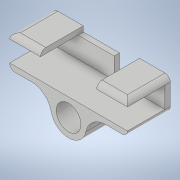
# Autodesk Inventor part: camera_holder
Saved by Autodesk Inventor 2020 (Build 240168000, 168)
## iProperties
Created: 2018-05-19
Part Number: camera_holder
Material: Generic
Document SubType Name: Modeling
Designer: stedrock
Density: 1 g/cm^3
Appearance: Default
Mass: 31.7935 g
Surface Area: 154.561 cm^2
Volume: 31.7935 cm^3
Author: stedrock
Autodesk Inventor part; units mm, degrees
ref_plane "YZ Plane" through (0, 0, 0) normal (1, 0, 0) x (0, 1, 0)
ref_plane "XZ Plane" through (0, 0, 0) normal (0, 1, 0) x (-1, 0, 0)
ref_plane "XY Plane" through (0, 0, 0) normal (0, 0, 1) x (1, 0, 0)
sketch "Sketch1" plane through (0, 0, 0) normal (0, 0, 1) x (1, 0, 0)
  line L0 (-44, -7.75) -> (44, -7.75)
  line L1 (44, -7.75) -> (44, 7.75)
  line L2 (44, 7.75) -> (-44, 7.75)
  line L3 (-44, 7.75) -> (-44, -7.75)
  line L4 (-44, -7.75) -> (44, 7.75) construction
  line L5 (44, -7.75) -> (-44, 7.75) construction
  line L6 (-44, -7.75) -> (44, -7.75)
  line L7 (44, -7.75) -> (44, -11.75)
  line L8 (44, -11.75) -> (-44, -11.75)
  line L9 (-44, -11.75) -> (-44, -7.75)
  line L10 (-44, 7.75) -> (-21, 7.75)
  line L11 (-21, 7.75) -> (-21, 11.75)
  line L12 (-21, 11.75) -> (-44, 11.75)
  line L13 (-44, 11.75) -> (-44, 7.75)
  line L14 (44, 7.75) -> (21, 7.75)
  line L15 (21, 7.75) -> (21, 11.75)
  line L16 (21, 11.75) -> (44, 11.75)
  line L17 (44, 11.75) -> (44, 7.75)
  line L18 (0, 0) -> (0, -41.0889) construction
  circle A0 centre (0, -21) radius 9.25
  circle A1 centre (0, -21) radius 13.25
  line L19 (-13.25, -21) -> (-13.25, -11.75)
  line L20 (-13.25, -11.75) -> (-9.4868, -11.75)
  line L21 (13.25, -11.75) -> (9.4868, -11.75)
  line L22 (13.25, -21) -> (13.25, -11.75)
  line L23 (13.25, -11.75) -> (9.4868, -11.75)
  line L24 (0, 0) -> (65.293, 0) construction
  line L25 (21, -7.75) -> (6, -7.75)
  line L26 (6, -7.75) -> (6, 7.75)
  line L27 (6, 7.75) -> (21, 7.75)
  line L28 (21, 7.75) -> (21, -7.75)
  line L29 (21, -7.75) -> (6, 7.75) construction
  line L30 (6, -7.75) -> (21, 7.75) construction
  point P0 (13.25, -21)
  point P1 (13.5, 0)
  dimension "d0" = 88
  dimension "d1" = 15.5
  dimension "d2" = 4
  dimension "d3" = 4
  dimension "d4" = 23
  dimension "d5" = 23
  dimension "d6" = 18.5
  dimension "d7" = 26.5
  dimension "d8" = 90
  dimension "d19" = 15
  dimension "d20" = 15.5
  dimension "d21" = 23
  constraints: 62 end point, 10 parallel, 6 horizontal, 6 point on line, 5 perpendicular, 4 midpoint, 4 point on circle, 2 centre point, 2 collinear, 2 symmetric about line, 2 tangent, 1 coincident, 1 vertical
  measures "d0" distance of L2.end L1.end
  measures "d1" distance of L1.end L0.end
  measures "d2" distance of L6.end L7.end
  measures "d3" distance of L12.end L2.end
  measures "d4" distance of L11.end L12.end
  measures "d5" distance of L15.end L16.end
  measures "d6" diameter of A0
  measures "d7" diameter of A1
  measures "d8" angle of L8 L19
  measures "d19" distance of L26.end L27.end
  measures "d20" distance of L25.end L26.end
  measures "d21" distance between parallel lines of L1 L28
extrude "main" add sketch "Sketch1" along normal blind 32 contours L0 L7 L8 A1 | A1 L8 L9 L0 | A1 L8 | L15 L16 L17 L2 | A1 L8 | L8 L22 A1 | A1 L19 L8 | L2 L13 L12 L11
extrude "bottom" add sketch "Sketch1" along normal blind 4 contours L0 L3 L2 L26 | L28 L2 L1 L0
fillet "Fillet1" radius 15 2 edges at (13.25, -11.75, 16) (-13.25, -11.75, 16)
fillet "Fillet2" radius 4 8 edges at (-44, 11.75, 16) (-44, -11.75, 16) (44, 11.75, 16) (44, -11.75, 16) (32.5, 11.75, 32) (-32.5, 11.75, 32) (21, -7.75, 2) (6, -7.75, 2)
equation "\"d2\" = wall"
equation "\"d3\" = wall2"
equation "\"d4\" = d5"
equation "\"d5\" = d21"
equation "\"d7\" = d6 + 2 * wall"
equation "\"d20\" = d1"
equation "\"d15\" = wall"
equation "\"d14\" = wall"
equation "\"wall\" = 4"
equation "\"wall2\" = 4"
body "Solid1"
